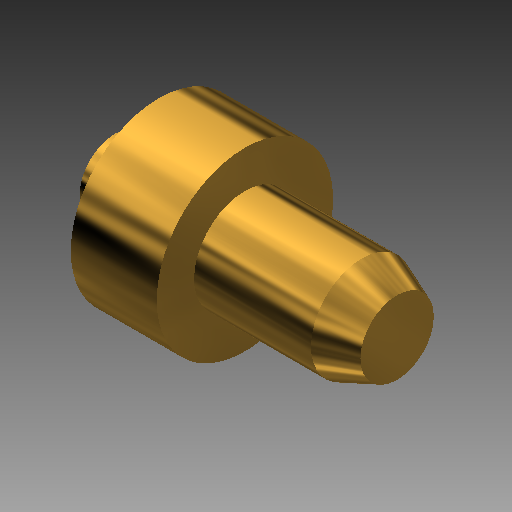
# Autodesk Inventor part: 403-04
Saved by Autodesk Inventor 2019 (Build 230136000, 136)
## iProperties
Company: Autodesk Inc.
Created: 2017-06-27
Part Number: 403-04
Material: Brass, Soft Yellow
Document SubType Name: Modeling
Designer: Autodesk Inc.
Mass: 0.662403 g
Surface Area: 1.20641 cm^2
Volume: 0.0782058 cm^3
Density: 8.47 g/cm^3
Appearance: Brass - Satin
Author: Inventor
Autodesk Inventor part; units mm, degrees
ref_plane "YZ Plane" through (0, 0, 0) normal (1, 0, 0) x (0, 1, 0)
ref_plane "XZ Plane" through (0, 0, 0) normal (0, 1, 0) x (-1, 0, 0)
ref_plane "XY Plane" through (0, 0, 0) normal (0, 0, 1) x (1, 0, 0)
sketch "Sketch1" plane through (0, 0, 0) normal (0, 0, 1) x (1, 0, 0)
  line L0 (0, 0) -> (1.25, 0)
  line L1 (1.25, 0) -> (1.25, 1)
  line L2 (1.25, 1) -> (0, 1)
  line L3 (0, 1) -> (0, 0)
  line L4 (1.25, 0) -> (3.685, 0)
  line L5 (3.685, 0) -> (3.685, 2.5)
  line L6 (3.685, 2.5) -> (1.25, 2.5)
  line L7 (1.25, 2.5) -> (1.25, 0)
  line L8 (3.685, 0) -> (8, 0)
  line L9 (8, 0) -> (8, 1.44)
  line L10 (8, 1.44) -> (3.685, 1.44)
  line L11 (3.685, 1.44) -> (3.685, 0)
  dimension "d0" = 1.25
  dimension "d1" = 3.685
  dimension "d2" = 8
  dimension "d3" = 2
  dimension "d4" = 5
  dimension "d5" = 2.88
  constraints: 24 end point, 6 parallel, 3 horizontal, 3 perpendicular
  measures "d0" distance of L2.end L1.end
  measures "d1" distance between parallel lines of L5 L3
  measures "d2" distance between parallel lines of L9 L3
  measures "d3" diameter of L2 L0
  measures "d4" diameter of L6 L8
  measures "d5" diameter of L10 L8
revolve "Revolution1" add sketch "Sketch1" angle 360 about axis through (3.685, 0, 0) along (1, 0, 0)
chamfer "Chamfer1" distance 0.4 distance2 1 1 edges at (8, -1.44, 0) measured on face at (8, -0.2568, -0.5255)
body "Solid1"
